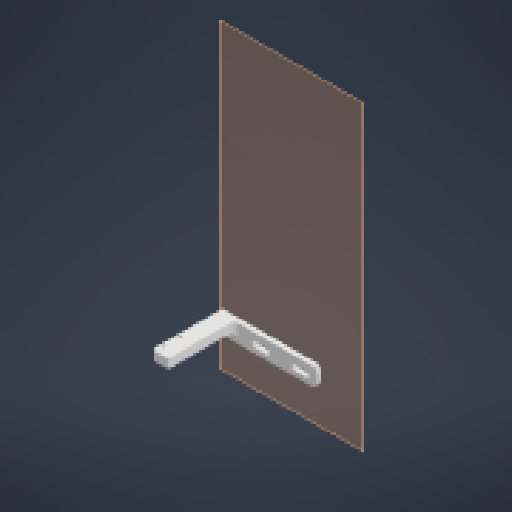
# Autodesk Inventor part: Homing_switch_holder
Saved by Autodesk Inventor 2026.1 (Build 301233020, 233B)
## iProperties
Created: 2025-11-05
Part Number: Homing_switch_holder
Material: Generic
Document SubType Name: Modeling
Designer: Mikke
Density: 1 g/cm^3
Appearance: Default
Author: Mikke
Autodesk Inventor part; units mm, degrees
ref_plane "YZ Plane" through (0, 0, 0) normal (1, 0, 0) x (0, 1, 0)
ref_plane "XZ Plane" through (0, 0, 0) normal (0, 1, 0) x (-1, 0, 0)
ref_plane "XY Plane" through (0, 0, 0) normal (0, 0, 1) x (1, 0, 0)
ref_plane "Work Plane1" through (0, 0, 0) normal (0, 0, 1) x (1, 0, 0)
sketch "Sketch1" plane through (0, 0, 0) normal (0, 0, 1) x (1, 0, 0)
  line L0 (18.2061, -59.3733) -> (-41.7939, -59.3733)
  line L1 (-41.7939, -59.3733) -> (-41.7939, -70.3733)
  line L2 (-41.7939, -70.3733) -> (18.2061, -70.3733)
  line L3 (18.2061, -70.3733) -> (18.2061, -59.3733)
  circle A0 centre (12, -65.5261) radius 1.75 projected
  circle A1 centre (-12, -65.5261) radius 1.75 projected
  line L4 (-12, -67.2761) -> (-12, -63.7761)
  line L5 (-12, -63.7761) -> (-19, -63.7761)
  line L6 (-19, -63.7761) -> (-19, -67.2761)
  line L7 (-19, -67.2761) -> (-12, -67.2761)
  line L8 (-12, -67.2761) -> (-12, -63.7761)
  line L9 (12, -67.2761) -> (12, -63.7761)
  line L10 (12, -63.7761) -> (5, -63.7761)
  line L11 (5, -63.7761) -> (5, -67.2761)
  line L12 (5, -67.2761) -> (12, -67.2761)
  line L13 (12, -67.2761) -> (12, -63.7761)
  circle A2 centre (-19, -65.5261) radius 1.75
  circle A3 centre (5, -65.5261) radius 1.75
  point P0 (0, 0)
  dimension "d0" = 60
  dimension "d1" = 11
  dimension "d13" = 7
  dimension "d14" = 7
  constraints: 28 end point, 6 parallel, 4 midpoint, 3 horizontal, 3 perpendicular, 2 vertical, 10 other
  measures "d0" distance of L0.start L0.end
  measures "d1" distance of L2.end L0.start
  measures "d13" distance of L7.end L6.end
  measures "d14" distance of L12.end L11.end
extrude "Extrusion1" add sketch "Sketch1" along normal blind 3
sketch "Sketch2" plane through (0, 0, 3) normal (0, 0, 1) x (1, 0, 0)
  line L0 (-41.7939, -59.3733) -> (-41.7939, -70.3733) projected
  line L1 (-41.7939, -59.3733) -> (-31.7939, -59.3733)
  line L2 (-31.7939, -59.3733) -> (-31.7939, -64.8733)
  line L3 (-31.7939, -64.8733) -> (-41.7939, -64.8733)
  line L4 (-41.7939, -64.8733) -> (-41.7939, -59.3733)
  point P0 (0, 0)
  dimension "d4" = 10
  dimension "d5" = 5.5
  constraints: 8 end point, 2 parallel, 1 horizontal, 1 perpendicular
  measures "d4" distance of L2.end L3.end
  measures "d5" distance of L1.end L2.end
extrude "Extrusion2" add sketch "Sketch2" along normal blind 40
sketch "Sketch3" plane through (-41.7939, -64.8733, 3) normal (0, -1, 0) x (1, 0, 0)
  circle A0 centre (2.0172, 35) radius 1.05 projected
  circle A1 centre (2.0172, 25) radius 1.05 projected
  point P0 (41.7939, -3)
extrude "Extrusion3" cut sketch "Sketch3" against normal blind 5.5
fillet "Fillet1" radius 1 2 edges at (-41.7939, -62.1233, 43) (-31.7939, -62.1233, 43)
fillet "Fillet2" radius 3 2 edges at (-36.7939, -64.8733, 3) (-31.7939, -62.1233, 3)
fillet "Fillet3" radius 3 3 edges at (18.2061, -59.3733, 1.5) (18.2061, -70.3733, 1.5) (-41.7939, -70.3733, 1.5)
body "Solid1"
